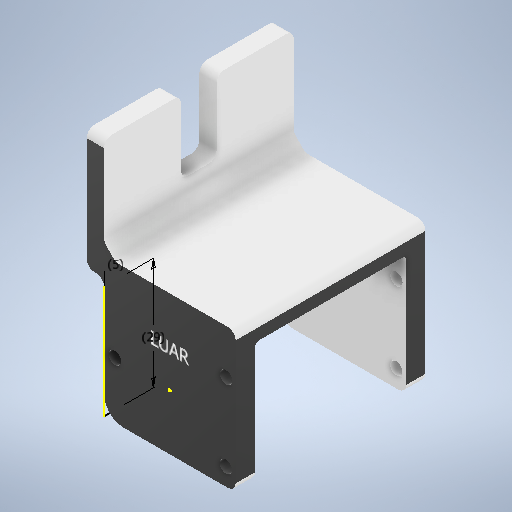
# Autodesk Inventor part: Part2
Saved by Autodesk Inventor 2025.1 (Build 291241000, 241)
## iProperties
Created: 2024-09-22
Part Number: Part2
Material: ABS Plastic
Document SubType Name: Modeling
Designer: JuhenFW
Density: 1.06 g/cm^3
Appearance: Smooth - White
Author: JuhenFW
Autodesk Inventor part; units mm, degrees
ref_plane "YZ Plane" through (0, 0, 0) normal (1, 0, 0) x (0, 1, 0)
ref_plane "XZ Plane" through (0, 0, 0) normal (0, 1, 0) x (-1, 0, 0)
sketch "Sketch1" plane through (0, 0, 0) normal (0, 0, 1) x (1, 0, 0)
  point P0 (0, 0)
sketch "Sketch2" plane through (0, 0, 0) normal (0, 0, 1) x (1, 0, 0)
  line L0 (-17, -14.5) -> (17, -14.5)
  line L1 (17, -14.5) -> (17, 14.5)
  line L2 (17, 14.5) -> (-17, 14.5)
  line L3 (-17, 14.5) -> (-17, -14.5)
  circle A0 centre (14.5, 10) radius 1.6
  circle A1 centre (14.5, -10) radius 1.6
  circle A2 centre (-14.2, 0) radius 1.6
  point P0 (0, 0)
  dimension "d0" = 34
  dimension "d1" = 29
  dimension "d2" = 3.2
  dimension "d3" = 3.2
  dimension "d4" = 3.2
  dimension "d5" = 20
  dimension "d6" = 2.5
  dimension "d7" = 14.5
  dimension "d8" = 28.7
  constraints: 8 end point, 3 centre point, 2 parallel, 1 horizontal, 1 perpendicular, 1 vertical alignment
  measures "d0" distance of L2.end L1.end
  measures "d1" distance between parallel lines of L0 L2
  measures "d2" diameter of A0
  measures "d3" diameter of A1
  measures "d4" diameter of A2
  measures "d5" distance of A1.centre A0.centre
  measures "d6" distance from line of L1 A1.centre
  measures "d7" distance from line of L2 A2.centre
  measures "d8" horizontal distance of A0.centre A2.centre
extrude "Extrusion1" add sketch "Sketch2" along normal blind 5
sketch "Sketch3" plane through (0, 0, 5) normal (0, 0, 1) x (1, 0, 0)
  line L0 (-7.3481, 13.6395) -> (7.272, 13.6395) construction
  line L1 (7.272, 13.6395) -> (7.272, 4.876) construction
  line L2 (7.272, 4.876) -> (-7.3481, 4.876) construction
  line L3 (-7.3481, 4.876) -> (-7.3481, 13.6395) construction
  point P0 (0, 0)
  constraints: 2 other
sketch "Sketch5" plane through (-17, -14.5, 0) normal (-1, 0, 0) x (0, 0, 1)
  line L0 (0, 0) -> (0, 29) projected
  line L1 (5, 0) -> (5, 29) projected
  line L2 (0, 29) -> (5, 29)
  line L3 (5, 29) -> (5, 0)
  line L4 (5, 0) -> (0, 0)
  line L5 (0, 0) -> (0, 29)
  point P0 (0, 14.5)
  dimension "d26" = 5
  dimension "d27" = 29
  constraints: 8 end point, 2 parallel, 1 horizontal, 1 perpendicular
  measures "d26" distance between parallel lines of L1 L0
  measures "d27" distance between parallel lines of L4 L2
sketch "Sketch6" plane through (-17, 14.5, 0) normal (0, 1, 0) x (1, 0, 0)
  line L0 (34, 0) -> (0, 0) projected
  line L1 (34, -5) -> (0, -5)
  line L2 (0, -5) -> (0, 0)
  line L3 (0, 0) -> (34, 0)
  line L4 (34, 0) -> (34, -5)
  point P0 (17, 0)
  dimension "d28" = 5
  dimension "d29" = 34
  constraints: 8 end point, 2 parallel, 1 horizontal, 1 perpendicular
  measures "d28" distance between parallel lines of L0 L1
  measures "d29" distance between parallel lines of L4 L2
extrude "Extrusion3" add sketch "Sketch6" along normal blind 2
sketch "Sketch7" plane through (-17, 16.5, 0) normal (0, 1, 0) x (1, 0, 0)
  line L0 (34, 0) -> (34, -5) projected
  line L1 (0, 0) -> (0, -5) projected
  line L2 (34, -5) -> (0, -5)
  line L3 (0, -5) -> (0, 0)
  line L4 (0, 0) -> (34, 0)
  line L5 (34, 0) -> (34, -5)
  point P0 (17, 0)
  constraints: 8 end point, 2 parallel, 1 horizontal, 1 perpendicular
extrude "Extrusion4" add sketch "Sketch7" along normal blind 5
sketch "Sketch8" plane through (0, 0, 0) normal (0, 0, -1) x (-1, 0, 0)
  line L0 (-17, -14.5) -> (-17, 21.5) projected
  line L1 (17, -14.5) -> (17, 21.5) projected
  line L2 (-17, 21.5) -> (17, 21.5)
  line L3 (17, 21.5) -> (17, 16.5)
  line L4 (17, 16.5) -> (-17, 16.5)
  line L5 (-17, 16.5) -> (-17, 21.5)
  point P0 (0, 0)
  dimension "d34" = 5
  constraints: 8 end point, 2 parallel, 1 horizontal, 1 perpendicular, 1 point on line
  measures "d34" distance between parallel lines of L4 L2
extrude "Extrusion5" add sketch "Sketch8" along normal blind 44
sketch "Sketch9" plane through (0, 0, 0) normal (0, 0, -1) x (-1, 0, 0)
  point P0 (0, 0)
ref_plane "Work Plane1" through (0, 0, -39) normal (0, 0, 1) x (1, 0, 0)
sketch "Sketch10" plane through (0, 0, -39) normal (0, 0, 1) x (1, 0, 0)
  circle A0 centre (14.5, -10) radius 1.6 projected
  circle A1 centre (14.5, -10) radius 1.6
  circle A2 centre (14.5, 10) radius 1.6 projected
  circle A3 centre (14.5, 10) radius 1.6
  circle A4 centre (-14.2, 0) radius 1.6 projected
  circle A5 centre (-14.2, 0) radius 1.6
  line L0 (-17, -14.5) -> (17, -14.5) projected
  line L1 (-17, -14.5) -> (-17, 21.5) projected
  line L2 (17, -14.5) -> (-17, -14.5)
  line L3 (-17, -14.5) -> (-17, 21.5)
  line L4 (-17, 21.5) -> (17, 21.5)
  line L5 (17, 21.5) -> (17, -14.5)
  point P0 (0, 0)
  dimension "d68" = 3.2
  dimension "d69" = 3.2
  dimension "d70" = 3.2
  constraints: 8 end point, 3 centre point, 3 coincident, 2 parallel, 1 horizontal, 1 perpendicular
  measures "d68" diameter of A3
  measures "d69" diameter of A5
  measures "d70" diameter of A1
extrude "Extrusion6" add sketch "Sketch10" against normal blind 5
sketch "Sketch16" plane through (0, 0, -39) normal (0, 0, 1) x (1, 0, 0)
  point P0 (0, 0)
sketch "Sketch17" plane through (-17, -14.5, 0) normal (-1, 0, 0) x (0, 0, 1)
  line L0 (-44, 36) -> (-44, 0) projected
  line L1 (5, 0) -> (5, 36) projected
  line L2 (-44, 36) -> (5, 36)
  line L3 (5, 36) -> (5, 31)
  line L4 (5, 31) -> (-44, 31)
  line L5 (-44, 31) -> (-44, 36)
  point P0 (0, 14.5)
  dimension "d42" = 5
  constraints: 8 end point, 2 parallel, 1 horizontal, 1 perpendicular, 1 point on line
  measures "d42" distance between parallel lines of L4 L2
extrude "Extrusion7" add sketch "Sketch17" along normal blind 4.5
sketch "Sketch18" plane through (-17, 21.5, 0) normal (0, 1, 0) x (1, 0, 0)
  line L0 (0, 44) -> (-4.5, 44) projected
  line L1 (0, -5) -> (34, -5) projected
  line L2 (-4.5, 44) -> (0, 44)
  line L3 (0, 44) -> (0, -5)
  line L4 (0, -5) -> (-4.5, -5)
  line L5 (-4.5, -5) -> (-4.5, 44)
  point P0 (17, 0)
  dimension "d45" = 4.5
  constraints: 8 end point, 2 parallel, 1 horizontal, 1 perpendicular
  measures "d45" distance between parallel lines of L5 L3
extrude "Extrusion8" add sketch "Sketch18" along normal blind 26
sketch "Sketch19" plane through (-21.5, -14.5, 0) normal (-1, 0, 0) x (0, 0, 1)
  line L0 (5, 31) -> (5, 62) projected
  line L1 (-44, 31) -> (-44, 62) projected
  line L2 (-44, 31) -> (5, 31) projected
  line L3 (-44, 62) -> (5, 62) projected
  line L4 (-44, 36) -> (-44, 62) projected
  line L5 (-44, 62) -> (-24.1, 62)
  line L6 (5, 62) -> (-14.9, 62)
  line L7 (-24.1, 62) -> (-14.9, 62)
  line L8 (-14.9, 62) -> (-14.9, 43)
  line L9 (-14.9, 43) -> (-24.1, 43)
  line L10 (-24.1, 43) -> (-24.1, 62)
  point P0 (0, 14.5)
  dimension "d48" = 49
  dimension "d49" = 31
  dimension "d50" = 19.9
  dimension "d51" = 19.9
  dimension "d52" = 19
  dimension "d79" = 9.2
  constraints: 12 end point, 2 parallel, 2 point on line, 1 horizontal, 1 perpendicular
  measures "d48" distance between parallel lines of L0 L1
  measures "d49" distance between parallel lines of L2 L3
  measures "d50" distance of L1.end L5.end
  measures "d51" distance of L0.end L6.end
  measures "d52" distance between parallel lines of L3 L9
  measures "d79" distance from line of L5.end L8
extrude "Extrusion9" cut sketch "Sketch19" against normal blind 26 contours L8 L9 L10 L3
fillet "Fillet1" radius 2 4 edges at (-19.25, 47.5, -24.1) (-19.25, 47.5, -14.9) (-19.25, 47.5, 5) (-19.25, 47.5, -44)
fillet "Fillet2" radius 2 2 edges at (-19.25, 28.5, -24.1) (-19.25, 28.5, -14.9)
fillet "Fillet3" radius 5 1 edges at (-17, -14.5, 2.5)
fillet "Fillet4" radius 5 1 edges at (-17, -14.5, -41.5)
fillet "Fillet5" radius 2 1 edges at (17, -14.5, 2.5)
fillet "Fillet6" radius 2 1 edges at (17, -14.5, -41.5)
fillet "Fillet7" radius 2 1 edges at (-21.5, 16.5, -19.5)
chamfer "Chamfer1" distance 3 angle 45 1 edges at (-17, 21.5, -19.5)
fillet "Fillet8" radius 2 2 edges at (-17, 24.5, -19.5) (-14, 21.5, -19.5)
fillet "Fillet9" radius 2 2 edges at (-17, 16.5, -41.5) (-17, 16.5, 2.5)
fillet "Fillet10" radius 2 1 edges at (17, 21.5, -19.5)
fillet "Fillet11" radius 1 2 edges at (-18, 16.5, 0) (0, 16.5, 0)
fillet "Fillet12" radius 1 1 edges at (0, 16.5, -39)
body "Solid1"
